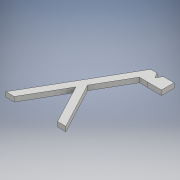
# Autodesk Inventor part: TableSupport
Saved by Autodesk Inventor 2018.3 (Build 223284000, 284)
## iProperties
Created: 2020-03-27
Part Number: TableSupport
Material: Generic
Document SubType Name: Modeling
Designer: Ivan
Density: 1 g/cm^3
Appearance: Default
Author: Ivan
Autodesk Inventor part; units mm, degrees
ref_plane "YZ Plane" through (0, 0, 0) normal (1, 0, 0) x (0, 1, 0)
ref_plane "XZ Plane" through (0, 0, 0) normal (0, 1, 0) x (-1, 0, 0)
ref_plane "XY Plane" through (0, 0, 0) normal (0, 0, 1) x (1, 0, 0)
sketch "Sketch1" plane through (0, 0, 0) normal (0, 0, 1) x (1, 0, 0)
  line L0 (0, 0) -> (55, 95.2628)
  line L1 (0, 0) -> (8.6603, 0)
  line L2 (64.8592, 0) -> (64.8592, 115) construction
  line L3 (64.8592, 0) -> (179.8592, 0) construction
  line L4 (56.1603, 82.2724) -> (65.4694, 82.2724) construction
  line L5 (79.2606, 82.2724) -> (79.2606, 95.2628)
  line L6 (55, 95.2628) -> (79.2606, 95.2628)
  line L7 (64.8592, 82.2724) -> (64.8592, 82.2824) construction
  line L8 (64.8592, 82.2824) -> (64.865, 82.2724)
  line L9 (64.8592, 82.2824) -> (64.8707, 82.2824) construction
  line L10 (64.8592, 82.2824) -> (64.8534, 82.2724)
  line L11 (64.8592, 82.2824) -> (64.8707, 82.2824) construction
  line L12 (64.865, 82.2724) -> (79.2606, 82.2724)
  line L13 (56.1603, 82.2724) -> (64.8534, 82.2724)
  line L14 (8.6603, 0) -> (53.6603, 0) construction
  line L15 (53.6603, 0) -> (32.0862, 40.5749)
  line L16 (53.6603, 0) -> (99.6142, 0) construction
  line L17 (36.5081, 48.2339) -> (62.1545, 0)
  line L18 (8.6603, 0) -> (32.0862, 40.5749)
  line L19 (36.5081, 48.2339) -> (56.1603, 82.2724)
  line L20 (62.1545, 0) -> (53.6603, 0)
  line L21 (79.2606, 95.2628) -> (79.2606, 82.2724) construction
  line L22 (64.8534, 82.2724) -> (64.865, 82.2724)
  dimension "d7" = 110
  dimension "d10" = 64.8592
  dimension "d11" = 115
  dimension "d12" = 90
  dimension "d15" = 95
  dimension "d22" = 0.01
  dimension "d23" = 60
  dimension "d24" = 120
  dimension "d27" = 45
  dimension "d28" = 118
  dimension "d29" = 7.5
  dimension "d43" = 7.5
  dimension "d44" = 7.5
  dimension "d45" = 24.2606
  dimension "d46" = 60
  constraints: 46 end point, 8 horizontal, 6 point on line, 4 equal length, 2 collinear, 2 parallel, 2 perpendicular, 2 vertical, 1 coincident
  measures "d7" distance of L0.start L0.end
  measures "d10" distance of L2.start L0.start
  measures "d11" distance of L2.start L2.end
  measures "d12" angle of L3 L2
  measures "d15" distance of L1.end L4.start
  measures "d22" distance of L7.start L7.end
  measures "d23" angle of L8 L9
  measures "d24" angle of L10 L11
  measures "d27" distance of L1.end L14.end
  measures "d28" angle of L16 L15
  measures "d29" distance between parallel lines of L15 L17
  measures "d43" distance between parallel lines of L19 L0
  measures "d44" distance between parallel lines of L0 L18
  measures "d45" distance of L0.end L5.end
  measures "d46" angle of L1 L18
extrude "Extrusion2" add sketch "Sketch1" along normal blind 5 contours L0 L6 L5 L12 L8 L10 L13 L19 L17 L20 L15 L18 L1
ref_plane "Work Plane2" through (64.8592, 82.2824, 5) normal (0.8660254, 0, 0.5) x (0, 1, 0)
ref_plane "Work Plane1" through (79.2606, 95.2628, 5) normal (0.8660254, 0, 0.5) x (0, 1, 0)
sketch "Sketch2" plane through (64.8592, 82.2824, 5) normal (0.8660254, 0, 0.5) x (0, 1, 0)
  line L0 (12.9804, -7.2007) -> (12.9804, 4.9296) construction
  line L1 (-0.01, 0.0029) -> (0, 0) construction
  line L2 (0, 0) -> (12.9804, 0) construction
  circle A0 centre (12.9804, 0) radius 2
  point P0 (-82.2824, 28.0995)
  dimension "d33" = 4
  constraints: 2 end point, 1 centre point, 1 coincident, 1 horizontal, 1 point on line
  measures "d33" diameter of A0
ref_plane "Work Plane3" through (64.8592, 82.2824, 5) normal (0.5, 0, -0.8660254) x (0, 1, 0)
sketch "Sketch3" plane through (64.8592, 82.2824, 5) normal (0.5, 0, -0.8660254) x (0, 1, 0)
  line L0 (-101.735, 0) -> (34.4329, 0) construction
  line L1 (12.9804, -11.0383) -> (12.9804, 9.972) construction
  line L2 (12.9804, 12.472) -> (12.9804, -8.5383) projected
  line L3 (12.9804, 0) -> (12.9804, 3)
  line L4 (12.9804, 3) -> (7.7842, 0)
  line L5 (7.7842, 0) -> (12.9804, -3)
  line L6 (12.9804, -3) -> (12.9804, 3)
  point P0 (-82.2824, -58.6697)
  dimension "d38" = 3
  dimension "d39" = 60
  dimension "d40" = 60
  constraints: 8 end point, 5 point on line, 1 collinear
  measures "d38" distance of L3.start L3.end
  measures "d39" angle of L4 L3
  measures "d40" angle of L5 L4
extrude "Extrusion4" cut sketch "Sketch3" along normal through all both and the other way through all
equation "\"d15\" = d7 - 2 * d9"
equation "\"d44\" = d43"
equation "\"d9\" = 7.5"
body "Solid2"
